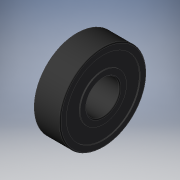
# Autodesk Inventor part: bearing_6000
Saved by Autodesk Inventor 2019 (Build 230136000, 136)
## iProperties
Created: 2023-11-09
Part Number: bearing_6000
Material: Generic
Catalog Web Link: www.cadenas.de
Description: 6000_bearing-Deep Groove Ball Bearings
Vendor: MISUMI
Document SubType Name: Modeling
Designer: psAdmin
Manufacturer: MISUMI
Mass: 3.45896 g
Surface Area: 18.5551 cm^2
Volume: 3.45896 cm^3
Density: 1 g/cm^3
Appearance: PSOLRGB-175-175-175
Category: PARTsolutions
Company: MISUMI
Title: bearing_6000
Author: Cadenas PARTsolutions
Comments: Deep Groove Ball Bearings
PSOL_IDENT_0: {$CADENAS_DATA/23d-libs/misumi/metric/accessories/bearing_6000.prj},170 {VTYP=3D},{NB=bearing_6000},
PSOL_IDENT_1: {LINA=bearing_6000},{NN=6000_bearing},{DATE=08.06.2021 06:39:28},{GEOMDATE=24.10.2013 00:00:00},{VER
PSOL_IDENT_2: SION=},{LINEID=40},{WBVAR=},{WBNUMERIC=}  {NB=bearing_6000},{LINA=bearing_6000},{KT=DUMMY},{PN=beari
PSOL_IDENT_3: ng_6000},{BN=6000},{DD=10},{D=26},{B=8},{RR=0.3},{DSMIN=12.0},{DS1=13.50},{DSMAX=13.50},{DDHH=24.0},
PSOL_IDENT_4: {R=0.3},{R1=0.200},{R2=0.300},{MASS=19},{MASS11=19},{AA=7.3380},{BB=1.9000},{CC=1.9500},{DD1=24.500}
NB: bearing_6000
NN: 6000_bearing
NT: Deep Groove Ball Bearings
NBSYN: $PN.
LINA: bearing_6000
CATALOG: Misumi
PN: bearing_6000
BN: 6000
DD: 10
D: 26
B: 8
RR: 0.3
DSMIN: 12
DDHH: 24
R: 0.3
MASS11: 19
SUPPLIER: MISUMI
ARTICLENO: bearing_6000
BOMINFO: bearing_6000
CREATOR: CADENAS GmbH
Autodesk Inventor part; units mm, degrees
sketch "Sketch_1" plane through (0, 0, 0) normal (0, 0, 1) x (1, 0, 0)
  line L0 (8, 0) -> (0, 0)
  arc A0 (0, 5.3) -> (0.3, 5) centre (0.3, 5.3) ccw
  line L1 (0.3, 5) -> (7.7, 5)
  arc A1 (7.7, 5) -> (8, 5.3) centre (7.7, 5.3) ccw
  line L2 (8, 5.3) -> (8, 6.95)
  line L3 (8, 6.95) -> (7.669, 6.95)
  line L4 (7.669, 6.95) -> (7.669, 11.1)
  line L5 (7.669, 11.1) -> (8, 11.1)
  line L6 (8, 11.1) -> (8, 12.7)
  arc A2 (8, 12.7) -> (7.7, 13) centre (7.7, 12.7) ccw
  line L7 (7.7, 13) -> (0.3, 13)
  arc A3 (0.3, 13) -> (0, 12.7) centre (0.3, 12.7) ccw
  line L8 (0, 12.7) -> (0, 11.1)
  line L9 (0, 11.1) -> (0.331, 11.1)
  line L10 (0.331, 11.1) -> (0.331, 6.95)
  line L11 (0.331, 6.95) -> (0, 6.95)
  line L12 (0, 6.95) -> (0, 5.3)
  constraints: 26 end point, 8 point on circle, 4 centre point
revolve "Revolution1" add sketch "Sketch_1" angle 360 about axis through (8, 0, 0) along (1, 0, 0)
ref_plane "center_point_XY" through (4, 0, 0) normal (1, 0, 0) x (0, 0, -1)
ref_plane "center_point_YZ" through (4, 0, 0) normal (0, 0, -1) x (0, 1, 0)
ref_plane "center_point_ZX" through (4, 0, 0) normal (0, 1, 0) x (1, 0, 0)
ref_plane "to_housing_XY" through (0, 0, 0) normal (1, 0, 0) x (0, 0, -1)
ref_plane "to_housing_YZ" through (0, 0, 0) normal (0, 0, -1) x (0, 1, 0)
ref_plane "to_housing_ZX" through (0, 0, 0) normal (0, 1, 0) x (1, 0, 0)
ref_plane "to_ring_XY" through (7.338, 0, 0) normal (1, 0, 0) x (0, 0, -1)
ref_plane "to_ring_YZ" through (7.338, 0, 0) normal (0, 0, -1) x (0, 1, 0)
ref_plane "to_ring_ZX" through (7.338, 0, 0) normal (0, 1, 0) x (1, 0, 0)
body "Solid1"
